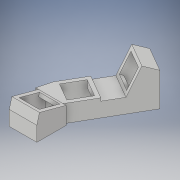
# Autodesk Inventor part: k2_thumb
Saved by Autodesk Inventor 2017 (Build 210142000, 142)
## iProperties
Created: 2017-02-06
Part Number: k2_thumb
Material: Generic
Document SubType Name: Modeling
Designer: herman
Density: 1 g/cm^3
Appearance: Default
Author: herman
Autodesk Inventor part; units mm, degrees
ref_plane "YZ Plane" through (0, 0, 0) normal (1, 0, 0) x (0, 1, 0)
ref_plane "XZ Plane" through (0, 0, 0) normal (0, 1, 0) x (-1, 0, 0)
ref_plane "XY Plane" through (0, 0, 0) normal (0, 0, 1) x (1, 0, 0)
sketch "Sketch1" plane through (0, 0, 0) normal (1, 0, 0) x (0, 1, 0)
  line L0 (1.6864, 14.4503) -> (11.8425, 14.4503)
  line L1 (11.8425, 14.4503) -> (18.604, 12.6385)
  line L2 (18.604, 12.6385) -> (13.6864, -5.714)
  line L3 (13.6864, -5.714) -> (1.6864, -5.714)
  line L4 (1.6864, -5.714) -> (1.6864, 14.4503)
  point P0 (0, 0)
  dimension "d0" = 19
  dimension "d1" = 7
  dimension "d2" = 105
  dimension "d3" = 12
  constraints: 10 end point, 2 perpendicular, 1 horizontal, 1 parallel
  measures "d0" distance of L1.end L2.end
  measures "d1" distance of L0.end L1.end
  measures "d2" angle of L3 L2
  measures "d3" distance of L2.end L3.end
extrude "Extrusion1" add sketch "Sketch1" along normal blind 19
sketch "Sketch2" plane through (0, 1.6864, -5.714) normal (0, -1, 0) x (1, 0, 0)
  line L0 (0, 0) -> (19, 0) projected
  line L1 (26.5, -16.4545) -> (10.0455, -25.9545)
  line L2 (0, 0) -> (0, 20.1643) construction
  line L3 (0.5455, -9.5) -> (10.0455, -25.9545)
  line L4 (-2, 0) -> (17, 0)
  line L5 (-2, 0) -> (0.5455, -9.5)
  line L6 (17, 0) -> (26.5, -16.4545)
  line L7 (17, 0) -> (0.5455, -9.5) construction
  point P0 (0, 5.714)
  dimension "d6" = 19
  dimension "d10" = 19
  dimension "d23" = 19
  dimension "d25" = 30
  dimension "d26" = 19
  dimension "d27" = 2
  constraints: 12 end point, 2 perpendicular, 1 horizontal, 1 point on line
  measures "d6" distance of L1.start L1.end
  measures "d10" distance of L3.start L1.end
  measures "d23" distance of L4.start L4.end
  measures "d25" angle of L7 L4
  measures "d26" distance of L4.end L1.start
  measures "d27" distance of L0.end L4.end
extrude "Extrusion2" add sketch "Sketch2" against normal blind 12
sketch "Sketch3" plane through (26.5, 1.6864, -22.1685) normal (0.8660254, 0, 0.5) x (0.5, 0, -0.8660254)
  line L0 (0, 0) -> (0, 10)
  line L1 (0, 10) -> (0, 15.9167) construction
  line L2 (0, 15.9167) -> (12.6883, 10) construction
  line L3 (12.6883, 10) -> (20.7181, 27.2198)
  line L4 (20.7181, 27.2198) -> (29.7811, 22.9937)
  line L5 (29.7811, 22.9937) -> (29.7811, 0)
  line L6 (29.7811, 0) -> (0, 0)
  line L7 (0, 10) -> (12.6883, 10)
  line L8 (0, 0) -> (0, 12) projected
  dimension "d16" = 19
  dimension "d17" = 10
  dimension "d18" = 14
  dimension "d20" = 25
  dimension "d30" = 10
  constraints: 16 end point, 5 perpendicular, 2 horizontal, 1 point on line
  measures "d16" distance of L2.end L3.end
  measures "d17" distance of L3.end L4.end
  measures "d18" distance of L1.end L2.end
  measures "d20" angle of L2 L7
  measures "d30" distance of L0.start L0.end
extrude "Extrusion4" add sketch "Sketch3" against normal blind 19
shell "Shell1" thickness 2.5 removed faces 1 at (27.7756, 1.6864, -37.0445)
sketch "Sketch4" plane through (0, 18.604, 12.6385) normal (0, 0.9659258, -0.258819) x (1, 0, 0)
  line L0 (2.5, 2.5) -> (16.5, 2.5) projected
  line L1 (16.5, 17.0817) -> (16.5, 2.5) projected
  line L2 (2.5, 2.5) -> (16.5, 2.5)
  line L3 (16.5, 2.5) -> (16.5, 17.0817)
  line L4 (16.5, 17.0817) -> (2.5, 17.0817)
  line L5 (2.5, 17.0817) -> (2.5, 2.5)
  point P0 (0, 17.023)
  constraints: 8 end point, 2 parallel, 1 horizontal, 1 perpendicular
sketch "Sketch5" plane through (0, 13.6864, -5.714) normal (0, 1, 0) x (1, 0, 0)
  line L0 (23.0849, 15.5394) -> (10.9606, 22.5394) projected
  line L1 (10.9606, 22.5394) -> (23.0849, 15.5394)
  line L2 (23.0849, 15.5394) -> (16.0849, 3.4151)
  line L3 (16.0849, 3.4151) -> (3.9606, 10.4151)
  line L4 (3.9606, 10.4151) -> (10.9606, 22.5394)
  point P0 (0, -5.714)
  dimension "d32" = 14
  constraints: 8 end point, 3 equal length, 1 perpendicular
  measures "d32" distance of L0.start L2.end
sketch "Sketch6" plane through (32.8442, 11.6864, -33.1569) normal (-0.4531539, 0.4226183, 0.7848856) x (0.8660254, 0, 0.5)
  line L0 (-16.5, 16.5) -> (-2.5, 16.5)
  line L1 (-2.5, 16.5) -> (-2.5, 2.5)
  line L2 (-2.5, 2.5) -> (-16.5, 2.5)
  line L3 (-16.5, 2.5) -> (-16.5, 16.5)
  line L4 (0, 19) -> (-19, 19) projected
  line L5 (-19, 0) -> (-19, 19) projected
  point P0 (-11.8654, -29.6671)
  dimension "d33" = 14
  dimension "d34" = 14
  dimension "d35" = 2.5
  dimension "d36" = 2.5
  constraints: 8 end point, 2 parallel, 1 horizontal, 1 perpendicular
  measures "d33" distance of L0.start L0.end
  measures "d34" distance of L2.end L0.start
  measures "d35" distance between parallel lines of L4 L0
  measures "d36" distance between parallel lines of L5 L3
extrude "Extrusion5" cut sketch "Sketch4" against normal up to next
extrude "Extrusion6" cut sketch "Sketch5" against normal up to next
extrude "Extrusion7" cut sketch "Sketch6" against normal up to next
body "Solid1"
